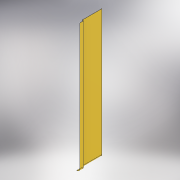
# Autodesk Inventor part: foil_shield
Saved by Autodesk Inventor 2020 (Build 240168000, 168)
## iProperties
Created: 2018-05-08
Part Number: foil_shield
Material: Generic
Document SubType Name: Modeling
Designer: PC  USER
Density: 1 g/cm^3
Appearance: Default
Author: PC  USER
Autodesk Inventor part; units mm, degrees
ref_plane "YZ Plane" through (0, 0, 0) normal (1, 0, 0) x (0, 1, 0)
ref_plane "XZ Plane" through (0, 0, 0) normal (0, 1, 0) x (-1, 0, 0)
ref_plane "XY Plane" through (0, 0, 0) normal (0, 0, 1) x (1, 0, 0)
sketch "Sketch1" plane through (0, 0, 0) normal (0, 1, 0) x (-1, 0, 0)
  line L0 (0, 0) -> (0, -97.227)
  line L1 (0, -97.227) -> (4.93, -97.227) construction
  arc A0 (0, -97.227) -> (4.93, -102.157) centre (4.93, -97.227) ccw
  line L2 (0.25, 0) -> (0.25, -97.227)
  arc A1 (0.25, -97.227) -> (4.93, -101.907) centre (4.93, -97.227) ccw
  line L3 (0.25, 0) -> (0, 0)
  line L4 (4.93, -101.907) -> (4.93, -102.157)
  dimension "d0" = 97.227
  dimension "d1" = 4.93
  dimension "d2" = 0.25
  constraints: 10 end point, 4 point on circle, 3 perpendicular, 2 centre point, 1 coincident, 1 vertical, 1 other
  measures "d0" distance of L0.start L0.end
  measures "d1" distance of L0.end L1.end
  measures "d2" distance between parallel lines of L0 L2
extrude "Extrusion1" add sketch "Sketch1" against normal blind 5.9
sketch "Sketch2" plane through (0, 0, 0) normal (0, 1, 0) x (1, 0, 0)
  arc A0 (-0.25, 97.227) -> (-4.93, 101.907) centre (-4.93, 97.227) ccw projected
  arc A1 (0, 97.227) -> (-4.93, 102.157) centre (-4.93, 97.227) ccw projected
  arc A2 (-1.97, 97.227) -> (-4.93, 100.187) centre (-4.93, 97.227) ccw
  line L0 (-1.97, 97.227) -> (-1.97, 0)
  line L1 (-1.97, 97.227) -> (95.257, 97.227) construction
  line L2 (-2.22, 0) -> (-2.22, 97.227)
  arc A3 (-2.22, 97.227) -> (-4.93, 99.937) centre (-4.93, 97.227) ccw
  line L3 (-2.22, 0) -> (-1.97, 0)
  line L4 (-4.93, 99.937) -> (-4.93, 100.187)
  point P0 (0, 0)
  dimension "d5" = 2.96
  dimension "d6" = 90
  dimension "d7" = 0.25
  constraints: 10 end point, 4 point on circle, 2 centre point, 2 horizontal, 2 perpendicular, 1 coincident, 1 other
  measures "d5" radius of A2
  measures "d6" angle of L0 L1
  measures "d7" distance between parallel lines of L0 L2
extrude "Extrusion2" add sketch "Sketch2" along normal blind 30
sketch "Sketch3" plane through (-0.25, 0, 0) normal (0, 0, 1) x (1, 0, 0)
  line L0 (-1.97, 0) -> (-1.72, 0) projected
  line L1 (-1.72, 0) -> (-1.72, 30) projected
  line L2 (-1.97, 30) -> (-1.72, 30) projected
  line L3 (-1.97, 0) -> (-1.97, 30) projected
  line L4 (0, 0) -> (0.25, 0) projected
  line L5 (0, 0) -> (0, -5.9) projected
  line L6 (0.25, -5.9) -> (0, -5.9) projected
  line L7 (0.25, 0) -> (0.25, -5.9) projected
  line L8 (0.25, 0) -> (-1.97, 0)
  line L9 (-1.97, 0) -> (-1.97, -0.25)
  line L10 (-1.97, -0.25) -> (0.25, -0.25)
  line L11 (0.25, -0.25) -> (0.25, 0)
  dimension "d10" = 0.25
  constraints: 8 end point, 2 parallel, 1 horizontal, 1 perpendicular
  measures "d10" distance of L9.end L8.end
sketch "Sketch4" plane through (0, 0, 0) normal (0, 1, 0) x (1, 0, 0)
  line L0 (-0.25, 97.227) -> (-0.25, 0) projected
  arc A0 (-0.25, 97.227) -> (-4.93, 101.907) centre (-4.93, 97.227) ccw projected
  point P0 (0, 0)
sketch3d "3D Sketch1"
  line L0 (-0.25, 0, 0) -> (-0.25, 0, -97.227)
  arc A0 (-0.25, 0, -97.227) -> (-4.93, 0, -101.907) centre (-4.93, 0, -97.227) ccw
sweep "Sweep1" add profiles "Sketch3" path "3D Sketch1" contours L0 L8 L5 L10 L9 | L4 L7 L10 L5
fillet "Fillet1" radius 0.4 4 edges at (-2.837, 0, -99.32) (-1.97, 0, -48.6135) (-1.444, 0, -100.713) (0, 0, -48.6135)
mirror "Mirror1" about plane through (0, 0, 0) normal (0, 0, 1) of "Fillet1", "Sweep1", "Extrusion2", "Extrusion1"
sketch "Sketch5" plane through (0, 30, 0) normal (0, 1, 0) x (1, 0, 0)
  line L0 (1.0174, -97.227) -> (-4.93, -97.227)
  line L1 (-4.93, -97.227) -> (-4.93, -102.8457)
  line L2 (-4.93, -102.8457) -> (1.0174, -102.8457)
  line L3 (1.0174, -102.8457) -> (1.0174, -97.227)
  line L4 (-0.4, -97.227) -> (0, -97.227) projected
  line L5 (-4.93, -101.757) -> (-4.93, -100.587) projected
  point P0 (0, 0)
  dimension "d14" = 0
  dimension "d15" = 0
  constraints: 8 end point, 2 parallel, 1 horizontal, 1 perpendicular
  measures "d14" distance between parallel lines of L0 L4
  measures "d15" distance between parallel lines of L5 L1
extrude "Extrusion3" cut sketch "Sketch5" against normal through all
body "Solid1"
